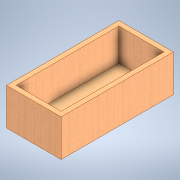
# Autodesk Inventor part: DarkBox
Saved by Autodesk Inventor 2022.2 (Build 262287010, 287A)
## iProperties
Created: 2022-05-02
Part Number: DarkBox
Material: Madera (cerezo)
Document SubType Name: Modeling
Designer: mabel
Density: 0.63 g/cm^3
Appearance: Cerezo - Natural brillo bajo
Author: mabel
Autodesk Inventor part; units mm, degrees
ref_plane "YZ Plane" through (0, 0, 0) normal (1, 0, 0) x (0, 1, 0)
ref_plane "XZ Plane" through (0, 0, 0) normal (0, 1, 0) x (-1, 0, 0)
ref_plane "XY Plane" through (0, 0, 0) normal (0, 0, 1) x (1, 0, 0)
sketch "Boceto1" plane through (0, 0, 0) normal (0, 1, 0) x (-1, 0, 0)
  line L0 (-85, -175) -> (85, -175)
  line L1 (85, -175) -> (85, 175)
  line L2 (85, 175) -> (-85, 175)
  line L3 (-85, 175) -> (-85, -175)
  line L4 (70, 160) -> (70, -160)
  line L5 (85, -160) -> (-85, -160)
  line L6 (-70, -160) -> (-70, 160)
  line L7 (-85, 160) -> (85, 160)
  line L8 (0, -160) -> (0, -60) construction
  line L9 (0, 175) -> (0, 29.19) construction
  circle A0 centre (0, 29.19) radius 5 construction
  line L10 (0, 29.19) -> (0, 0.69) construction
  line L11 (0, 29.19) -> (0, 57.69) construction
  line L12 (17.8997, 57.69) -> (-17.8997, 57.69) construction
  line L13 (-17.8997, 57.69) -> (-17.8997, 0.69) construction
  line L14 (-17.8997, 0.69) -> (17.8997, 0.69) construction
  line L15 (17.8997, 0.69) -> (17.8997, 57.69) construction
  point P0 (0, 0)
  dimension "d0" = 170
  dimension "d1" = 350
  dimension "d2" = 15
  dimension "d7" = 100
  dimension "d8" = 145.81
  dimension "d9" = 10
  dimension "d12" = 28.5
  dimension "d13" = 28.5
  constraints: 32 end point, 9 point on line, 6 parallel, 3 perpendicular, 3 vertical, 2 horizontal, 2 midpoint, 1 centre point, 1 coincident
  measures "d0" distance of L2.end L1.end
  measures "d1" distance of L1.end L0.end
  measures "d2" distance between parallel lines of L1 L4
  measures "d7" distance of L8.start L8.end
  measures "d8" distance of L9.start L9.end
  measures "d9" diameter of A0
  measures "d12" distance of L10.start L10.end
  measures "d13" distance of L10.start L11.end
extrude "Extrusión1" add sketch "Boceto1" along normal blind 100 contours L3 L5 L1 L0
extrude "Extrusión2" add sketch "Boceto1" along normal blind 100 contours L5 L4 L7 L1
extrude "Extrusión3" add sketch "Boceto1" against normal blind 15
sketch "Boceto2" plane through (-70, 100, -160) normal (0, 0, 1) x (1, 0, 0)
  line L0 (155, -100) -> (155, 0) construction
  line L1 (0, 0) -> (77.5, 0)
  line L2 (0, 0) -> (155, 0) projected
  line L3 (77.5, -100) -> (70, -100) construction
  line L4 (0, -100) -> (155, -100) construction
  line L5 (70, -100) -> (70, -74.5) construction
  circle A0 centre (70, -74.5) radius 2.5
  circle A1 centre (70, -74.5) radius 7.5
  dimension "d94" = 7.5
  dimension "d95" = 25.5
  dimension "d96" = 5
  dimension "d97" = 5
  constraints: 6 end point, 2 centre point, 1 coincident, 1 midpoint, 1 point on line
  measures "d94" distance of L3.start L3.end
  measures "d95" distance of L3.end L5.end
  measures "d96" diameter of A0
  measures "d97" radial gap between concentric circles of A0 A1
extrude "Extrusión4" cut sketch "Boceto2" against normal through all contours A0
extrude "Extrusión5" add sketch "Boceto1" along normal blind 100 contours L3 L2 L1 L7
extrude "Extrusión6" add sketch "Boceto1" along normal blind 100 contours L3 L7 L6 L5
sketch "Boceto3" plane through (0, 0, 0) normal (0, 1, 0) x (1, 0, 0)
  line L0 (-70, -160) -> (-70, 160) construction
  line L1 (-70, -160) -> (7.5, -160) construction
  line L2 (-70, -160) -> (85, -160) construction
  line L3 (-70, -160) -> (7.5, -160) construction
  line L4 (7.5, -29.19) -> (-9, -29.19) construction
  line L5 (15, -57.69) -> (5.97, -57.69)
  line L6 (5.97, -57.69) -> (5.97, -48.59)
  line L7 (5.97, -48.59) -> (15, -48.59)
  line L8 (15, -48.59) -> (15, -57.69)
  line L9 (15, -0.69) -> (7.47, -0.69)
  line L10 (7.47, -0.69) -> (7.47, -13.65)
  line L11 (7.47, -13.65) -> (15, -13.65)
  line L12 (15, -13.65) -> (15, -0.69)
  line L13 (85, 175) -> (85, -175) projected
  line L14 (85, -29.19) -> (0, -29.19) construction
  circle A0 centre (0, -29.19) radius 3.5
  line L15 (0, -29.19) -> (0, -22.225) construction
  line L16 (-15, -57.69) -> (-5.97, -57.69)
  line L17 (-5.97, -48.59) -> (-15, -48.59)
  line L18 (-15, -48.59) -> (-15, -57.69)
  line L19 (-15, -0.69) -> (-7.47, -0.69)
  line L20 (-7.47, -0.69) -> (-7.47, -13.65)
  line L21 (-7.47, -13.65) -> (-15, -13.65)
  line L22 (-15, -13.65) -> (-15, -0.69)
  line L23 (-5.97, -57.69) -> (-5.97, -48.59)
  line L24 (-85, -175) -> (85, -175) projected
  point P0 (-85, -160)
  point P1 (15, -7.17)
  point P2 (-15, -7.17)
  dimension "d46" = 9.03
  dimension "d47" = 9.1
  dimension "d48" = 12.96
  dimension "d54" = 85
  dimension "d55" = 7
  dimension "d62" = 30
  dimension "d63" = 30
  dimension "d68" = 70
  dimension "d69" = 117.31
  dimension "d70" = 90.97
  dimension "d71" = 161.35
  dimension "d72" = 70
  dimension "d73" = 7.53
  dimension "d74" = 92.47
  constraints: 42 end point, 8 symmetric about line, 5 equal length, 3 horizontal, 3 midpoint, 2 perpendicular, 2 point on line, 2 vertical, 1 centre point, 1 coincident
  measures "d46" distance of L6.end L7.end
  measures "d47" distance of L5.end L6.end
  measures "d48" distance of L10.end L9.end
  measures "d54" distance of L14.start L14.end
  measures "d55" diameter of A0
  measures "d62" distance of point (15, -7.17) point (-15, -7.17)
  measures "d63" distance between parallel lines of L8 L18
  measures "d68" distance between parallel lines of L13 L8
  measures "d69" distance between parallel lines of L24 L5
  measures "d70" distance between parallel lines of L13 L23
  measures "d71" distance between parallel lines of L24 L11
  measures "d72" distance between parallel lines of L13 L12
  measures "d73" distance of L9.start L9.end
  measures "d74" distance between parallel lines of L13 L20
extrude "Extrusión12" cut sketch "Boceto3" against normal blind 5 contours L5 L6 L7 L8 | L12 L11 L10 L9 | L18 L17 L23 L16 | L19 L20 L21 L22
extrude "Extrusión13" cut sketch "Boceto3" against normal through all contours A0
sketch "Boceto8" plane through (85, 100, -160) normal (1, 0, 0) x (0, 0, -1)
  line L0 (-320, -100) -> (0, -100) projected
  line L1 (0, -100) -> (-100, -100)
  line L2 (-100, -100) -> (-100, -14.2875)
  line L3 (-335, -100) -> (0, -100) projected
  line L4 (-192.69, -100) -> (-185.69, -100) projected
  line L5 (-189.19, -100) -> (-100, -100)
  line L6 (-335, -115) -> (15, -115) projected
  point P0 (-160, -100)
  dimension "d66" = 100
  dimension "d67" = 89.19
  constraints: 6 end point, 1 midpoint, 1 parallel, 1 perpendicular, 1 point on line
  measures "d66" distance of L0.end L1.end
  measures "d67" distance from line of L5.start L2
sketch "Boceto9" plane through (0, 0, 0) normal (0, 1, 0) x (1, 0, 0)
  line L0 (0, 160) -> (0, 60)
  line L1 (0, 60) -> (40, 60) construction
  line L2 (0, 60) -> (-40, 60) construction
  line L3 (0, 60) -> (-40, 60) construction
  line L4 (40, 60) -> (40, 52.5) construction
  line L5 (40, 60) -> (40, 67.5) construction
  line L6 (40, 67.5) -> (20, 67.5)
  line L7 (20, 67.5) -> (20, 52.5)
  line L8 (20, 52.5) -> (40, 52.5)
  line L9 (40, 52.5) -> (40, 67.5)
  line L10 (-40, 60) -> (-40, 67.5) construction
  line L11 (-40, 67.5) -> (-20, 67.5)
  line L12 (-20, 67.5) -> (-20, 52.5)
  line L13 (-20, 52.5) -> (-40, 52.5)
  line L14 (-40, 67.5) -> (-40, 52.5)
  line L15 (-20, 80) -> (-40, 80)
  line L16 (-40, 80) -> (-40, 40)
  line L17 (-40, 40) -> (-20, 40)
  line L18 (-20, 40) -> (-20, 80)
  line L19 (20, 80) -> (40, 80)
  line L20 (40, 80) -> (40, 40)
  line L21 (40, 40) -> (20, 40)
  line L22 (20, 40) -> (20, 80)
  point P0 (0, 0)
  point P1 (-30, 60)
  dimension "d80" = 100
  dimension "d83" = 40
  dimension "d86" = 7.5
  dimension "d87" = 7.5
  dimension "d88" = 20
  dimension "d89" = 15
  dimension "d98" = 20
  dimension "d99" = 40
  constraints: 46 end point, 8 symmetric about line, 4 horizontal, 4 parallel, 3 perpendicular, 1 collinear, 1 point on line, 1 vertical
  measures "d80" distance of L0.start L0.end
  measures "d83" distance of L0.end L2.end
  measures "d86" distance of L1.end L4.end
  measures "d87" distance of L1.end L5.end
  measures "d88" distance of L8.end L7.end
  measures "d89" distance of L7.end L6.end
  measures "d98" distance of L17.end L16.end
  measures "d99" distance of L16.end L15.end
extrude "Extrusión14" [suppressed]
sketch "Boceto10" plane through (0, 0, 0) normal (0, 1, 0) x (1, 0, 0)
  circle A0 centre (0, -29.19) radius 3.5 projected
  line L0 (0, -29.19) -> (0, 170.81)
  line L1 (0, -29.19) -> (200, -29.19) construction
  point P0 (0, 0)
  dimension "d92" = 200
  dimension "d93" = 90
  constraints: 4 end point, 1 horizontal, 1 perpendicular, 1 vertical
  measures "d92" distance of L0.start L0.end
  measures "d93" angle of L1 L0
extrude "Extrusión15" [suppressed]
